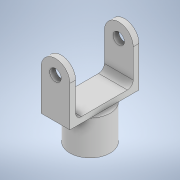
# Autodesk Inventor part: uJoint.1
Saved by Autodesk Inventor 2021 (Build 250183000, 183)
## iProperties
Created: 2022-04-15
Part Number: uJoint.1
Material: Generic
Document SubType Name: Modeling
Designer: Łukasz
Density: 1 g/cm^3
Appearance: Default
Author: Łukasz
Autodesk Inventor part; units mm, degrees
ref_plane "YZ Plane" through (0, 0, 0) normal (1, 0, 0) x (0, 1, 0)
ref_plane "XZ Plane" through (0, 0, 0) normal (0, 1, 0) x (-1, 0, 0)
ref_plane "XY Plane" through (0, 0, 0) normal (0, 0, 1) x (1, 0, 0)
sketch "Sketch1" plane through (0, 0, 0) normal (0, 0, 1) x (1, 0, 0)
  circle A0 centre (0, 0) radius 5
  circle A1 centre (0, 0) radius 12.5
  line L0 (-12.5, 0) -> (12.5, 0)
  line L1 (12.5, 0) -> (12.5, -30)
  line L2 (12.5, -30) -> (-12.5, -30)
  line L3 (-12.5, -30) -> (-12.5, 0)
  dimension "d1" = 25
  dimension "d0" = 10
  dimension "d2" = 25
  dimension "d3" = 30
  constraints: 8 end point, 2 coincident, 2 parallel, 1 centre point, 1 horizontal, 1 perpendicular, 3 other
  measures "d0" diameter of A0
  measures "d2" distance of L1.end L2.end
  measures "d3" distance of L0.end L1.end
extrude "Extrusion1" add sketch "Sketch1" along normal blind 5 contours L0 A1 A0 | A0 L0 A1 | L1 L2 L3 A1
pattern_linear "Rectangular Pattern1" count 2 spacing 55 along (0, 0, 1) of "Extrusion1"
sketch "Sketch2" plane through (-12.5, -30, 55) normal (0, -1, 0) x (1, 0, 0)
  line L0 (0, 5) -> (25, 5) projected
  line L1 (25, 5) -> (0, 5)
  line L2 (0, 5) -> (0, -55)
  line L3 (0, -55) -> (25, -55)
  line L4 (25, -55) -> (25, 5)
  point P0 (12.5, -55)
  constraints: 8 end point, 2 parallel, 1 horizontal, 1 perpendicular
extrude "Extrusion2" add sketch "Sketch2" along normal blind 5
fillet "Fillet1" radius 5 2 edges at (0, -30, 5) (0, -30, 55)
sketch "Sketch3" plane through (-12.5, -35, 55) normal (0, -1, 0) x (1, 0, 0)
  circle A0 centre (12.5, -25) radius 17.5
  circle A1 centre (12.5, -25) radius 12.5
  line L0 (0, -55) -> (25, -55) projected
  point P0 (12.5, -55)
  dimension "d12" = 35
  dimension "d15" = 30
  constraints: 2 centre point, 1 coincident
  measures "d12" diameter of A0
  measures "d15" distance from line of L0 A0.centre
extrude "Extrusion3" add sketch "Sketch3" along normal blind 30
body "Solid1"
